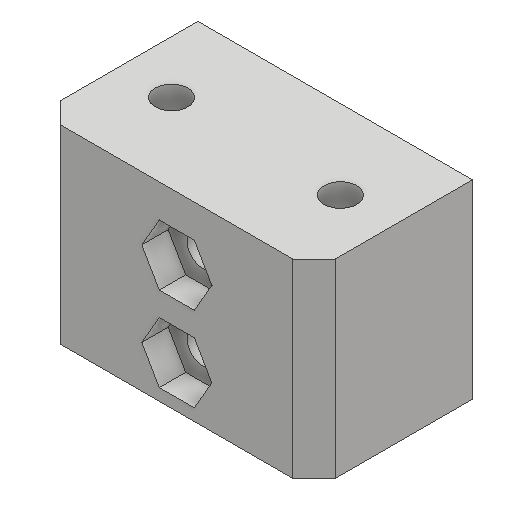
# Autodesk Inventor part: 3DP_ABS_Z_Axis_IGUS_Cable_Chain_Mount
Saved by Autodesk Inventor 2026.1 (Build 301233000, 233)
## iProperties
Created: 2016-06-21
Part Number: 3DP_ABS_Z_Axis_IGUS_Cable_Chain_Mount
Material: Ogólny
Document SubType Name: Modeling
Designer: Andrzej
Density: 1 g/cm^3
Appearance: Domyślna
Mass: 6.48147 g
Surface Area: 27.7131 cm^2
Volume: 6.48147 cm^3
Author: Andrzej
Autodesk Inventor part; units mm, degrees
ref_plane "YZ Plane" through (0, 0, 0) normal (1, 0, 0) x (0, 1, 0)
ref_plane "XZ Plane" through (0, 0, 0) normal (0, 1, 0) x (-1, 0, 0)
ref_plane "XY Plane" through (0, 0, 0) normal (0, 0, 1) x (1, 0, 0)
sketch "Szkic1" plane through (0, 0, 0) normal (0, 0, 1) x (1, 0, 0)
  line L0 (-7.8594, 6.1623) -> (18.1406, 6.1623)
  line L1 (18.1406, 6.1623) -> (18.1406, -8.8377)
  line L2 (18.1406, -8.8377) -> (-7.8594, -8.8377)
  line L3 (-7.8594, -8.8377) -> (-7.8594, 6.1623)
  point P0 (0, 0)
  point P1 (-2.8594, -1.3377)
  point P2 (13.1406, -1.3377)
  dimension "d0" = 26
  dimension "d1" = 15
  dimension "d4" = 7.5
  dimension "d5" = 7.5
  dimension "d6" = 5
  dimension "d7" = 5
  constraints: 8 end point, 2 parallel, 1 horizontal, 1 perpendicular
  measures "d0" distance of L1.end L2.end
  measures "d1" distance of L0.end L1.end
  measures "d4" distance from line of L2 point (-2.859, -1.338)
  measures "d5" distance from line of L2 point (13.141, -1.338)
  measures "d6" distance from line of L3 point (-2.859, -1.338)
  measures "d7" distance from line of L1 point (13.141, -1.338)
extrude "Wyciągnięcie proste1" add sketch "Szkic1" along normal blind 18
hole "Otwór1" at (-2.8594, -1.3377, 0) at (13.1406, -1.3377, 0) direction (0, 0, 1) diameter 3.1 end through all
sketch "Szkic2" plane through (-7.8594, -8.8377, 0) normal (0, -1, 0) x (1, 0, 0)
  line L0 (26, 0) -> (0, 0) projected
  line L1 (26, 0) -> (26, 18) projected
  line L2 (0, 18) -> (26, 18) projected
  line L3 (0, 0) -> (0, 18) projected
  point P0 (7.8594, 0)
  point P1 (13, 12)
  point P2 (13, 4)
  dimension "d16" = 8
  dimension "d17" = 13
  dimension "d18" = 26
  dimension "d19" = 13
  dimension "d27" = 4
  measures "d16" distance of point (13, 12) point (13, 4)
  measures "d17" distance from line of L3 point (13, 12)
  measures "d18" distance of L2.start L1.end
  measures "d19" distance from line of L3 point (13, 4)
  measures "d27" distance from line of L0 point (13, 4)
hole "Otwór2" at (5.1406, -8.8377, 12) at (5.1406, -8.8377, 4) direction (0, 1, 0) diameter 3.1 end through all
chamfer "Faza2" distance 2 angle 45 2 edges at (-7.8594, -8.8377, 9) (18.1406, -8.8377, 9)
sketch "Szkic4" plane through (-5.8594, -8.8377, 0) normal (0, -1, 0) x (1, 0, 0)
  line L0 (22, 18) -> (22, 0) projected
  line L1 (0, 18) -> (22, 18) projected
  line L2 (0, 0) -> (0, 18) projected
  line L3 (22, 0) -> (0, 0) projected
  circle A0 centre (11, 12) radius 1.55 projected
  circle A1 centre (11, 4) radius 1.55 projected
  line L4 (12.6599, 14.875) -> (14.3198, 12)
  line L5 (14.3198, 12) -> (12.6599, 9.125)
  line L6 (12.6599, 9.125) -> (9.3401, 9.125)
  line L7 (9.3401, 9.125) -> (7.6802, 12)
  line L8 (7.6802, 12) -> (9.3401, 14.875)
  line L9 (9.3401, 14.875) -> (12.6599, 14.875)
  line L10 (12.6599, 6.875) -> (14.3198, 4)
  line L11 (14.3198, 4) -> (12.6599, 1.125)
  line L12 (12.6599, 1.125) -> (9.3401, 1.125)
  line L13 (9.3401, 1.125) -> (7.6802, 4)
  line L14 (7.6802, 4) -> (9.3401, 6.875)
  line L15 (9.3401, 6.875) -> (12.6599, 6.875)
  point P0 (5.8594, 0)
  point P1 (11, 14.875)
  point P2 (11, 6.875)
  constraints: 24 end point, 2 midpoint, 26 other
extrude "Wyciągnięcie proste3" cut sketch "Szkic4" against normal blind 2.5 contours L4 L5 L6 L7 L8 L9 | L10 L11 L12 L13 L14 L15
equation "\"d4\" = 0.5 * d1"
equation "\"d5\" = d4"
equation "\"d17\" = 0.5 * d18"
equation "\"d19\" = d17"
